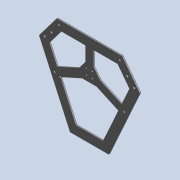
# Autodesk Inventor part: ChestMount
Saved by Autodesk Inventor 2020 (Build 240168000, 168)
## iProperties
Created: 2021-08-03
Part Number: ChestMount
Material: Generic
Document SubType Name: Sheet Metal
Designer: Val
Density: 1 g/cm^3
Sheet Metal Rule: Default
Appearance: Default
Author: Val
Autodesk Inventor part; units mm, degrees
ref_plane "YZ Plane" through (0, 0, 0) normal (1, 0, 0) x (0, 1, 0)
ref_plane "XZ Plane" through (0, 0, 0) normal (0, 1, 0) x (-1, 0, 0)
ref_plane "XY Plane" through (0, 0, 0) normal (0, 0, 1) x (1, 0, 0)
sketch "Base" plane through (0, 0, 0) normal (0, 0, 1) x (1, 0, 0)
  circle A0 centre (12.1878, 3.2978) radius 3.175
  circle A1 centre (-5.7727, -14.6627) radius 3.175
  circle A2 centre (212.3944, 3.2978) radius 3.175
  circle A3 centre (230.3549, -14.6627) radius 3.175
  arc A4 (-21.1681, -17.0473) -> (9.6227, 23.6429) centre (-130.3641, 97.5775) ccw construction
  arc A5 (214.9596, 23.6429) -> (245.7503, -17.0473) centre (354.9463, 97.5775) ccw construction
  line L0 (26.2432, 41.3978) -> (-19.9769, -19.6825)
  line L1 (12.1878, 3.2978) -> (212.3944, 3.2978) construction
  line L2 (112.2911, 41.3978) -> (112.2911, -199.9022) construction
  line L3 (26.2432, 41.3978) -> (112.2911, 41.3978)
  line L4 (-19.9769, -19.6825) -> (61.4911, -199.9022)
  line L5 (61.4911, -199.9022) -> (112.2911, -199.9022)
  line L6 (9.6227, 23.6429) -> (-21.1681, -17.0473) construction
  line L7 (-19.9769, -19.6825) -> (-21.1681, -17.0473) construction
  line L8 (62.3467, -158.4118) -> (162.2358, -158.4118) construction
  line L9 (89.4311, 18.5378) -> (89.4311, -177.0422) construction
  line L10 (89.4311, -177.0422) -> (76.2445, -177.0422)
  line L11 (76.2445, -177.0422) -> (6.4492, -22.6443)
  line L12 (6.4492, -22.6443) -> (37.6121, 18.5378)
  line L13 (37.6121, 18.5378) -> (89.4311, 18.5378)
  line L14 (89.4311, 18.5378) -> (112.2911, 18.5378)
  line L15 (89.4311, -177.0422) -> (112.2911, -177.0422)
  line L16 (198.339, 41.3978) -> (244.5591, -19.6825)
  line L17 (198.339, 41.3978) -> (112.2911, 41.3978)
  line L18 (244.5591, -19.6825) -> (163.0911, -199.9022)
  line L19 (163.0911, -199.9022) -> (112.2911, -199.9022)
  line L20 (135.1511, -177.0422) -> (148.3377, -177.0422)
  line L21 (148.3377, -177.0422) -> (218.133, -22.6443)
  line L22 (218.133, -22.6443) -> (186.9701, 18.5378)
  line L23 (186.9701, 18.5378) -> (135.1511, 18.5378)
  line L24 (135.1511, 18.5378) -> (112.2911, 18.5378)
  line L25 (135.1511, -177.0422) -> (112.2911, -177.0422)
  point P0 (0, 0)
  point P1 (112.2911, 3.2978)
extrude "Plate1" add sketch "Base" along normal blind 3.048
sketch "Sketch2" plane through (0, 0, 3.048) normal (0, 0, 1) x (1, 0, 0)
  circle A0 centre (104.2911, -48.2622) radius 2.05
  circle A1 centre (104.2911, -32.2622) radius 2.05
  circle A2 centre (120.2911, -32.2622) radius 2.05
  circle A3 centre (120.2911, -48.2622) radius 2.05
  line L0 (120.2911, -32.2622) -> (104.2911, -32.2622) construction
  line L1 (104.2911, -32.2622) -> (104.2911, -48.2622) construction
  line L2 (104.2911, -48.2622) -> (120.2911, -48.2622) construction
  line L3 (120.2911, -48.2622) -> (120.2911, -32.2622) construction
  line L4 (186.9701, 18.5378) -> (37.6121, 18.5378)
  line L5 (148.3377, -177.0422) -> (76.2445, -177.0422)
  line L6 (112.2911, 18.5378) -> (112.2911, -177.0422) construction
  line L7 (76.2445, -177.0422) -> (148.3377, -177.0422)
  line L8 (122.4511, 18.5378) -> (122.4511, -19.5622)
  line L9 (122.4511, -19.5622) -> (139.7677, -42.4462)
  line L10 (139.7677, -42.4462) -> (197.4038, -68.5005)
  line L11 (218.133, -22.6443) -> (148.3377, -177.0422)
  line L12 (189.0337, -87.0165) -> (131.3975, -60.9622)
  line L13 (131.3975, -60.9622) -> (112.2911, -60.9622)
  line L14 (218.133, -22.6443) -> (186.9701, 18.5378)
  line L15 (148.3377, -177.0422) -> (218.133, -22.6443)
  line L16 (122.4511, -19.5622) -> (112.2911, -19.5622) construction
  line L17 (139.7677, -42.4462) -> (131.3975, -60.9622) construction
  line L18 (102.1311, 18.5378) -> (102.1311, -19.5622)
  line L19 (102.1311, -19.5622) -> (84.8146, -42.4462)
  line L20 (84.8146, -42.4462) -> (27.1784, -68.5005)
  line L21 (35.5486, -87.0165) -> (93.1847, -60.9622)
  line L22 (93.1847, -60.9622) -> (112.2911, -60.9622)
  line L23 (122.4511, 18.5378) -> (102.1311, 18.5378)
  line L24 (197.4038, -68.5005) -> (189.0337, -87.0165)
  line L25 (27.1784, -68.5005) -> (35.5486, -87.0165)
  line L26 (76.2445, -177.0422) -> (6.4492, -22.6443)
  point P0 (0, 0)
  point P1 (112.2911, -32.2622)
  dimension "d8" = 16
  dimension "d9" = 16
  dimension "d10" = 50.8
  dimension "d11" = 10.16
  dimension "d12" = 20.32
  dimension "d13" = 12.7
  dimension "d14" = 12.7
  measures "d8" distance of L0.start L0.end
  measures "d9" distance of L0.end L1.end
  measures "d10" distance between parallel lines of L0 L4
  measures "d11" distance between parallel lines of L6 L8
  measures "d12" distance between parallel lines of L12 L10
  measures "d13" distance between parallel lines of L16 L0
  measures "d14" distance between parallel lines of L2 L13
sheet face with bend "Face2" sketch "Sketch2" thickness 3.048 toward (0, 0, -1) bend radius 3.048 relief straight relief width 3.048 relief depth 1.524 contours L8 L9 L10 L11 L12 L13 L22 L21 L25 L20 L19 L18 L4
bend "Bend1"
sketch "Sketch3" plane through (0, 0, 3.048) normal (0, 0, 1) x (1, 0, 0)
  circle A0 centre (31.9277, 29.9678) radius 2.794
  line L0 (26.2432, 41.3978) -> (-19.9769, -19.6825) projected
  line L1 (6.4492, -22.6443) -> (37.6121, 18.5378) projected
  line L2 (26.2432, 41.3978) -> (37.6121, 18.5378) construction
  line L3 (186.9701, 18.5378) -> (218.133, -22.6443) projected
  line L4 (244.5591, -19.6825) -> (198.339, 41.3978) projected
  line L5 (186.9701, 18.5378) -> (198.339, 41.3978) construction
  circle A1 centre (192.6545, 29.9678) radius 2.794
  line L6 (27.1784, -68.5005) -> (6.4492, -22.6443) projected
  line L7 (27.1784, -68.5005) -> (35.5486, -87.0165) construction
  line L8 (31.3635, -77.7585) -> (10.533, -87.1749) construction
  line L9 (61.4911, -199.9022) -> (-19.9769, -19.6825) projected
  circle A2 centre (20.9482, -82.4667) radius 2.794
  line L10 (26.2432, 41.3978) -> (198.339, 41.3978) projected
  line L11 (112.2911, 41.3978) -> (112.2911, -60.9622) construction
  line L12 (93.1847, -60.9622) -> (131.3975, -60.9622) projected
  circle A3 centre (203.634, -82.4667) radius 2.794
  point P0 (0, 0)
  dimension "d20" = 5.588
  dimension "d21" = 5.588
  constraints: 10 end point, 6 midpoint, 4 centre point, 2 coincident, 1 equal radius, 1 perpendicular, 1 point on line, 1 symmetric about line, 1 other
  measures "d20" diameter of A0
  measures "d21" diameter of A2
hole "Hole1" at (31.9277, 29.9678, 3.048) at (192.6545, 29.9678, 3.048) at (20.9482, -82.4667, 3.048) at (203.634, -82.4667, 3.048) direction (0, 0, -1) diameter 5.588 end through all
equation "\"d12\" = 2 * d11"
equation "\"d27\" = Thickness"
equation "\"d7\" = Thickness"
equation "\"d15\" = BendRadius"
equation "\"d16\" = BendReliefWidth"
equation "\"d18\" = MinimumRemnant"
equation "\"d17\" = BendReliefDepth"
equation "\"d19\" = TransitionRadius"
equation "\"BendRadius\" = Thickness"
equation "\"BendReliefWidth\" = Thickness"
equation "\"BendReliefDepth\" = 0.5 * Thickness"
equation "\"CornerReliefSize\" = 4 * Thickness"
equation "\"MinimumRemnant\" = 2 * Thickness"
equation "\"TransitionRadius\" = BendRadius"
equation "\"JacobiRadiusSize\" = BendRadius"
equation "\"GapSize\" = Thickness"
equation "\"Thickness\" = 3.048"
body "Solid1"
